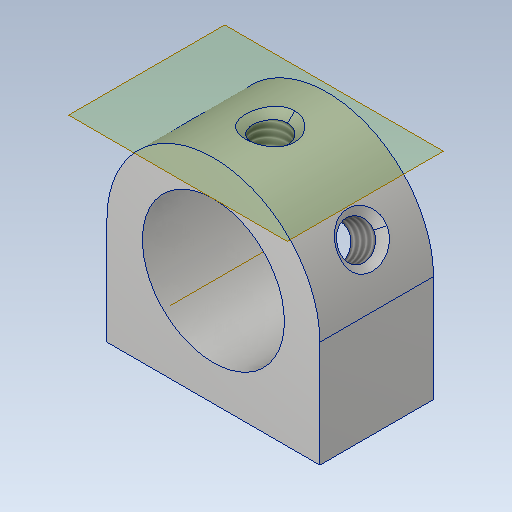
# Autodesk Inventor part: LowerArm_Shaft_Fixation
Saved by Autodesk Inventor 2021.4 (Build 254397000, 397)
## iProperties
Created: 2022-07-05
Part Number: LowerArm_Shaft_Fixation
Material: Aluminum 6061
Document SubType Name: Modeling
Designer: alexw
Density: 2.7 g/cm^3
Appearance: Aluminum - Flat
Mass: 2.50529 g
Surface Area: 9.77782 cm^2
Volume: 0.927883 cm^3
ShaftFixation_Width: 15,000 mm
ShaftFixataion_Hole_Dist: 10,500 mm
ShaftFixation_Height: 15,000 mm
Author: alexw
Autodesk Inventor part; units mm, degrees
note: some values were not read from the file. Chosen so that the rebuilt part matches the saved one: direction of "Hole1".
ref_plane "YZ Plane" through (0, 0, 0) normal (1, 0, 0) x (0, 1, 0)
ref_plane "XZ Plane" through (0, 0, 0) normal (0, 1, 0) x (-1, 0, 0)
ref_plane "XY Plane" through (0, 0, 0) normal (0, 0, 1) x (1, 0, 0)
sketch "Sketch1" plane through (0, 0, 0) normal (0, 0, 1) x (1, 0, 0)
  circle A0 centre (0, 7.5) radius 5
  circle A1 centre (0, 7.5) radius 7.5 construction
  line L0 (-10.5, 0) -> (10.5, 0) construction
  line L1 (7.5, 1.8) -> (-7.5, 1.8) construction
  line L2 (-7.5, 7.5) -> (-7.5, 0)
  line L3 (7.5, 7.5) -> (7.5, 0)
  line L4 (0, 0) -> (0, 7.5) construction
  arc A2 (7.5, 7.5) -> (-7.5, 7.5) centre (0, 7.5) ccw
  line L5 (-7.5, 0) -> (7.5, 0)
  point P0 (0, 15)
  dimension "d0" = 10
  dimension "d1" = 2.5
  dimension "d3" = 15
  dimension "d4" = 1.8
  dimension "ShaftFixation_Width" = 15
  dimension "ShaftFixation_Height" = 15
  constraints: 10 end point, 5 point on circle, 4 point on line, 4 tangent, 3 centre point, 2 perpendicular, 1 coincident, 1 collinear, 1 vertical
  measures "d0" diameter of A0
  measures "d1" radial gap between concentric circles of A0 A1
  measures "d3" diameter of A1
  measures "d4" distance between parallel lines of L0 L1
  measures "ShaftFixation_Width" distance between parallel lines of L3 L2
  measures "ShaftFixation_Height" distance from line of L0 point (0, 15)
extrude "Extrusion1" add sketch "Sketch1" along normal blind 8
ref_plane "Work Plane1" through (0, 15, 0) normal (0, -1, 0) x (1, 0, 0)
sketch "Sketch2" plane through (0, 15, 0) normal (0, -1, 0) x (1, 0, 0)
  line L0 (0, 0) -> (0, 8) construction
  point P0 (0, 4)
  constraints: 1 midpoint
hole "Hole1" at (0, 15, 4) direction (0, -1, 0) diameter 2.459 end up to surface thread size "M3x0.5" class "6H" standard "ISO Metric profile"
pattern_circular "Circular Pattern1" count 2 over 60 about axis through (0, 7.5, 0) along (0, 0, 1) of "Hole1"
pattern_circular "Circular Pattern2" count 2 over 60 about axis through (0, 7.5, 0) along (0, 0, -1) of "Hole1"
chamfer "Chamfer1" distance 0.5 angle 45 6 edges at (-5.7926, 12.264, 4.0016) (-7.0221, 10.1345, 4.0003) (1.2295, 14.8985, 4.0016) (-1.2295, 14.8985, 4.0003) (7.0221, 10.1345, 4.0016) (5.7926, 12.264, 4.0003)
sketch "Sketch4" plane through (-7.5, 0, 0) normal (0, -1, 0) x (1, 0, 0)
  line L0 (0, 0) -> (0, 8) construction
  line L1 (0, 4) -> (15, 4) construction
  line L2 (15, 0) -> (15, 8) construction
  line L3 (7.5, -1.6) -> (7.5, 9.6) construction
  point P0 (7.5, 0)
  point P1 (2.25, 4)
  point P2 (12.75, 4)
  dimension "d32" = 5.25
  dimension "ShaftFixataion_Hole_Dist" = 10.5
  constraints: 2 end point, 2 midpoint, 1 point on line, 1 symmetric about line
  measures "d32" distance from line of point (2.25, 4) L3
  measures "ShaftFixataion_Hole_Dist" distance of point (12.75, 4) point (2.25, 4)
hole "Hole3" at (-5.25, 0, 4) at (5.25, 0, 4) direction (0, 1, 0) diameter 1.567 depth 3 tip angle 118 thread size "M2x0.4" class "6H" standard "ISO Metric profile"
equation "\"d0\" = Shaft_DiaOut"
equation "\"Shaft_DiaOut\" = 10"
body "Solid1"
